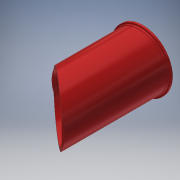
# Autodesk Inventor part: A1-19010-200-02 HCWI nozzle insert
Saved by Autodesk Inventor 2017.3 (Build 213257000, 257)
## iProperties
Created: 2014-07-18
Part Number: A1-19010-200-02 HCWI nozzle insert
Material: Iron, Cast
Document SubType Name: Modeling
Designer: Graeme_Van_Dongen
Density: 7.25 g/cm^3
Appearance: Light Red
Description: 30" HCWI NOZZLE, ASTM A532 CLASS III TYPE A, PF# 741280
Mass: 540851 g
Surface Area: 47359.6 cm^2
Volume: 74600.2 cm^3
Author: Graeme_Van_Dongen
Autodesk Inventor part; units mm, degrees
ref_plane "YZ Plane" through (0, 0, 0) normal (1, 0, 0) x (0, 1, 0)
ref_plane "XZ Plane" through (0, 0, 0) normal (0, 1, 0) x (-1, 0, 0)
ref_plane "XY Plane" through (0, 0, 0) normal (0, 0, 1) x (1, 0, 0)
sketch "Sketch1" plane through (0, 0, 0) normal (0, 0, 1) x (1, 0, 0)
  circle A0 centre (0, 0) radius 374.904
  dimension "d0" = 749.808
  constraints: 1 centre point, 1 coincident
  measures "d0" diameter of A0
extrude "Extrusion1" add sketch "Sketch1" along normal blind 25.4
sketch "Sketch2" plane through (0, 0, 0) normal (0, 0, 1) x (1, 0, 0)
  circle A0 centre (0, 0) radius 355.854
  dimension "d3" = 711.708
  constraints: 1 centre point, 1 coincident
  measures "d3" diameter of A0
extrude "Extrusion2" add sketch "Sketch2" along normal blind 50
sketch "Sketch3" plane through (0, 0, 0) normal (0, 0, 1) x (1, 0, 0)
  circle A0 centre (0, 0) radius 349.25
  dimension "d6" = 698.5
  constraints: 1 centre point, 1 coincident
  measures "d6" diameter of A0
extrude "Extrusion3" add sketch "Sketch3" along normal blind 1330.7314
sketch "Sketch4" plane through (0, 0, 1330.7314) normal (0, 0, 1) x (1, 0, 0)
  circle A0 centre (-6.35, 0) radius 317.5
  point P0 (0, 0)
  dimension "d9" = 635
  dimension "d21" = 6.35
  constraints: 1 centre point, 1 horizontal alignment
  measures "d9" diameter of A0
  measures "d21" distance of point (0, 0) A0.centre
extrude "Extrusion4" cut sketch "Sketch4" against normal through all
chamfer "Chamfer1" distance 0.7937 angle 45 1 edges at (-374.904, 0, 25.4)
fillet "Fillet1" radius 0.7937 1 edges at (-355.854, 0, 25.4)
fillet "Fillet2" radius 0.7937 1 edges at (-349.25, 0, 50)
sketch "Sketch5" plane through (0, 0, 0) normal (0, 1, 0) x (-1, 0, 0)
  line L0 (-311.15, 1330.7314) -> (323.85, 1330.7314) projected
  line L1 (-311.15, 1330.7314) -> (323.85, 797.9031)
  line L2 (323.85, 797.9031) -> (349.25, 797.9031)
  line L3 (349.25, 797.9031) -> (349.25, 1330.7314)
  line L4 (349.25, 1330.7314) -> (323.85, 1330.7314)
  line L5 (349.25, 50.7937) -> (349.25, 1330.7314) construction
  point P0 (0, 0)
  dimension "d18" = 40
  constraints: 8 end point, 2 perpendicular, 1 collinear, 1 parallel, 1 vertical alignment
  measures "d18" angle of L0 L1
extrude "Extrusion5" cut sketch "Sketch5" along normal through all both and the other way through all
body "Solid1"
